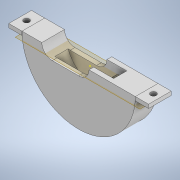
# Autodesk Inventor part: Деталь56
Saved by Autodesk Inventor 2022 (Build 260153000, 153)
## iProperties
Created: 2023-02-08
Part Number: Деталь56
Material: Типовые
Document SubType Name: Modeling
Designer: 89160908988
Density: 1 g/cm^3
Appearance: По умолчанию
Author: 89160908988
Autodesk Inventor part; units mm, degrees
ref_plane "YZ Plane" through (0, 0, 0) normal (1, 0, 0) x (0, 1, 0)
ref_plane "XY Plane" through (0, 0, 0) normal (0, 0, 1) x (1, 0, 0)
sketch "Эскиз1" plane through (0, 0, 0) normal (0, 0, 1) x (1, 0, 0)
  circle A0 centre (0, 0) radius 762
  dimension "d0" = 1524
  constraints: 1 centre point, 1 coincident
  measures "d0" diameter of A0
extrude "Выдавливание1" add sketch "Эскиз1" along normal mid plane 304.8
sketch "Эскиз2" plane through (0, 0, 0) normal (0, 0, 1) x (1, 0, 0)
  circle A0 centre (0, 0) radius 406.4
  dimension "d3" = 812.8
  constraints: 1 centre point, 1 coincident
  measures "d3" diameter of A0
extrude "Выдавливание2" cut sketch "Эскиз2" along normal mid plane 177.8
ref_plane "РабПлоскость1" through (0, -101.6, 0) normal (0, 1, 0) x (-1, 0, 0)
sketch "Эскиз3" plane through (0, -101.6, 0) normal (0, 1, 0) x (-1, 0, 0)
  line L0 (406.4, 88.9) -> (-406.4, 88.9) projected
  line L1 (-406.4, -88.9) -> (406.4, -88.9) projected
  line L2 (-406.4, 88.9) -> (-279.4, 88.9)
  line L3 (-279.4, 88.9) -> (-279.4, -88.9)
  line L4 (-279.4, -88.9) -> (-406.4, -88.9)
  line L5 (-406.4, -88.9) -> (-406.4, 88.9)
  point P0 (0, 0)
  dimension "d7" = 127
  constraints: 8 end point, 2 parallel, 1 horizontal, 1 perpendicular, 1 point on line
  measures "d7" distance between parallel lines of L5 L3
extrude "Выдавливание3" add sketch "Эскиз3" against normal blind 177.8
sketch "Эскиз4" plane through (0, 0, 152.4) normal (0, 0, 1) x (1, 0, 0)
  line L0 (0, 0) -> (-355.6, 0) construction
  line L1 (0, -139.7) -> (-355.6, -139.7)
  line L2 (-355.6, 139.7) -> (0, 139.7)
  arc A0 (0, -139.7) -> (0, 139.7) centre (0, 0) ccw
  arc A1 (-355.6, 139.7) -> (-355.6, -139.7) centre (-355.6, 0) ccw
  point P0 (-177.8, 0)
  dimension "d10" = 355.6
  dimension "d11" = 279.4
  constraints: 8 end point, 4 point on circle, 4 tangent, 2 centre point, 1 horizontal, 1 midpoint, 1 parallel
  measures "d10" distance of L0.start L0.end
  measures "d11" distance between parallel lines of L1 L2
extrude "Выдавливание4" cut sketch "Эскиз4" against normal through all
sketch "Эскиз5" plane through (0, 0, 0) normal (0, 1, 0) x (-1, 0, 0)
  line L0 (762, 152.4) -> (-762, 152.4) projected
  line L1 (-762, -152.4) -> (762, -152.4) projected
  line L2 (762, 152.4) -> (-762, 152.4)
  line L3 (-762, 152.4) -> (-762, -152.4)
  line L4 (-762, -152.4) -> (762, -152.4)
  line L5 (762, -152.4) -> (762, 152.4)
  point P0 (0, 0)
  constraints: 8 end point, 2 parallel, 1 horizontal, 1 perpendicular
extrude "Выдавливание5" cut sketch "Эскиз5" along normal blind 762
sketch "Эскиз6" plane through (0, 0, 0) normal (0, 1, 0) x (-1, 0, 0)
  line L0 (-762, -152.4) -> (-762, 152.4) projected
  line L1 (-762, -152.4) -> (-939.8, -152.4)
  line L2 (-939.8, -152.4) -> (-939.8, 152.4)
  line L3 (-939.8, 152.4) -> (-762, 152.4)
  line L4 (-762, 152.4) -> (-762, -152.4)
  line L5 (0, 447.1525) -> (0, -527.7865)
  line L6 (-762, 152.4) -> (-139.7, 152.4) projected
  line L7 (-139.7, -152.4) -> (-762, -152.4) projected
  line L8 (762, -152.4) -> (762, 152.4)
  line L9 (762, -152.4) -> (939.8, -152.4)
  line L10 (939.8, -152.4) -> (939.8, 152.4)
  line L11 (939.8, 152.4) -> (762, 152.4)
  point P0 (0, 0)
  dimension "d16" = 304.8
  dimension "d17" = 177.8
  constraints: 18 end point, 5 symmetric about line, 2 collinear, 2 parallel, 1 horizontal, 1 perpendicular, 1 point on line, 1 vertical
  measures "d16" distance between parallel lines of L3 L1
  measures "d17" distance between parallel lines of L2 L0
extrude "Выдавливание6" add sketch "Эскиз6" against normal blind 50.8
sketch "Эскиз7" plane through (0, -101.6, 0) normal (0, 1, 0) x (-1, 0, 0)
  point P0 (0, 0)
sketch "Эскиз8" plane through (0, 0, 0) normal (0, 1, 0) x (-1, 0, 0)
  circle A0 centre (852.8874, 0) radius 38.1
  line L0 (0, 193.2199) -> (0, -225.4232)
  circle A1 centre (-852.8874, 0) radius 38.1
  point P0 (0, 0)
  dimension "d20" = 76.2
  constraints: 2 centre point, 2 end point, 1 point on line, 1 symmetric about line, 1 vertical, 1 other
  measures "d20" diameter of A0
extrude "Выдавливание7" cut sketch "Эскиз8" against normal through all
